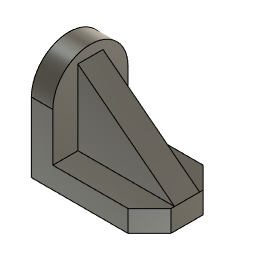
A1 (Autodesk Fusion 360 design; units mm, degrees)
Autodesk Fusion 360 part; units mm, degrees
sketch "Base" plane through (0, 0, 0) normal (0, 0, 1) x (1, 0, 0)
  line L0 (0, 0) -> (66, 0)
  line L1 (66, 0) -> (66, 42)
  line L2 (66, 42) -> (0, 42)
  line L3 (0, 42) -> (0, 0)
  dimension "d17" = 42
  dimension "d18" = 66
  constraint horizontal L0
  constraint vertical L1
  constraint horizontal L2
  constraint vertical L3
  constraint coincident L0.start L3.end
  measures "d17" distance of L0.start L2.end
  measures "d18" distance of L0.start L0.end
extrude "Extrude4" add sketch "Base" along normal blind 12
chamfer "Chamfer1" distance 12 angle 45 2 edges at (66, 42, 6) (66, 0, 6)
sketch "Body" plane through (0, 0, 12) normal (0, 0, 1) x (-1, 0, 0)
  line L0 (-54, 0) -> (-66, -12)
  line L1 (-66, -12) -> (-66, -30)
  line L2 (-66, -30) -> (-54, -42)
  line L3 (-54, -42) -> (0, -42)
  line L4 (0, -42) -> (0, 0)
  line L5 (0, 0) -> (-54, 0)
  line L6 (0, 0) -> (-12, 0)
  line L7 (-12, 0) -> (-12, -42)
  line L8 (-12, -42) -> (0, -42)
  line L9 (0, -42) -> (0, 0)
  dimension "d22" = 12
  dimension "d23" = 42
  constraint horizontal L6
  constraint vertical L7
  constraint horizontal L8
  constraint vertical L9
  constraint coincident L4.end L5.start
  measures "d22" distance of L4.end L6.end
  measures "d23" distance of L4.end L3.end
extrude "Extrude5" add sketch "Body" along normal blind 48 contours L3 L4 L5 L6 L7 L8 L9
fillet "Fillet1" radius 21 2 edges at (6, 42, 60) (6, 0, 60)
sketch "Triangle" plane through (0, 0, 0) normal (0, 1, 0) x (1, 0, 0)
  line L0 (66, -12, 21) -> (12, -12, 21)
  line L1 (12, -12, 21) -> (12, -54, 21)
  line L2 (12, -54, 21) -> (66, -12, 21)
extrude "Extrude6" add sketch "Triangle" along normal mid plane 14 contours L0 L1 L2 in plane through (0, 21, 0) normal (0, 1, 0)
equation "d24 = 60 mm - 12 mm"
named bodies: "Object"
